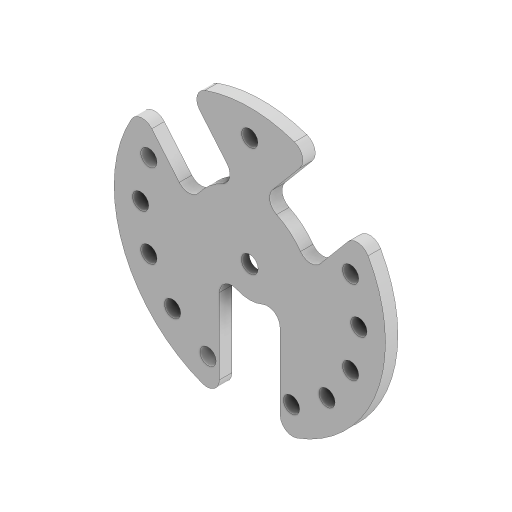
# Autodesk Inventor part: LED disk
Saved by Autodesk Inventor 2024 (Build 280153000, 153)
## iProperties
Created: 2025-04-26
Part Number: LED disk
Material: Generic
Document SubType Name: Modeling
Designer: Binara
Density: 1 g/cm^3
Appearance: Default
Author: Binara
## iProperties of the stored document LED disk_3DPrint.ipt
Created: 2025-04-26
Part Number: LED disk_3DPrint
Material: Generic
Document SubType Name: Modeling
Designer: Binara
Density: 1 g/cm^3
Appearance: Default
Author: Binara
Autodesk Inventor part; units mm, degrees
ref_plane "YZ Plane" through (0, 0, 0) normal (1, 0, 0) x (0, 1, 0)
ref_plane "XZ Plane" through (0, 0, 0) normal (0, 1, 0) x (-1, 0, 0)
ref_plane "XY Plane" through (0, 0, 0) normal (0, 0, 1) x (1, 0, 0)
sketch "Sketch1" plane through (0, 0, 0) normal (0, 0, 1) x (1, 0, 0)
  circle A0 centre (0, 0) radius 43.5
  circle A1 centre (0, 35) radius 2.6
  circle A2 centre (-13.3939, 32.3358) radius 2.6
  circle A3 centre (-24.7487, 24.7487) radius 2.6
  circle A4 centre (-32.3358, 13.3939) radius 2.6
  circle A5 centre (-35, 0) radius 2.6
  circle A6 centre (-32.3358, -13.3939) radius 2.6
  circle A7 centre (-24.7487, -24.7487) radius 2.6
  circle A8 centre (-13.3939, -32.3358) radius 2.6
  circle A9 centre (0, -35) radius 2.6
  circle A10 centre (13.3939, -32.3358) radius 2.6
  circle A11 centre (24.7487, -24.7487) radius 2.6
  circle A12 centre (32.3358, -13.3939) radius 2.6
  circle A13 centre (35, 0) radius 2.6
  circle A14 centre (32.3358, 13.3939) radius 2.6
  circle A15 centre (24.7487, 24.7487) radius 2.6
  circle A16 centre (13.3939, 32.3358) radius 2.6
  line L0 (0, 0) -> (0, -92.2535) construction
  line L1 (-9.7254, 0) -> (-9.7254, -92.2535)
  line L2 (9.7254, -92.2535) -> (9.7254, 0)
  arc A17 (9.7254, 0) -> (-9.7254, 0) centre (0, 0) ccw
  arc A18 (-9.7254, -92.2535) -> (9.7254, -92.2535) centre (0, -92.2535) ccw
  line L3 (0, 0) -> (-60.6432, 72.2718) construction
  line L4 (-7.6604, -6.4279) -> (-68.3037, 65.8439)
  line L5 (-52.9828, 78.6997) -> (7.6604, 6.4279)
  arc A19 (-7.6604, -6.4279) -> (7.6604, 6.4279) centre (0, 0) ccw
  arc A20 (-52.9828, 78.6997) -> (-68.3037, 65.8439) centre (-60.6432, 72.2718) ccw
  line L6 (0, 0) -> (65.9097, 78.5481) construction
  line L7 (-7.6604, 6.4279) -> (58.2493, 84.976)
  line L8 (73.5702, 72.1203) -> (7.6604, -6.4279)
  arc A21 (-7.6604, 6.4279) -> (7.6604, -6.4279) centre (0, 0) ccw
  arc A22 (73.5702, 72.1203) -> (58.2493, 84.976) centre (65.9097, 78.5481) ccw
  circle A23 centre (0, 0) radius 20
  point P0 (0, -46.1267)
  point P1 (-30.3216, 36.1359)
  point P2 (32.9549, 39.2741)
  point P3 (18.7939, 6.8404)
  point P4 (3.473, 19.6962)
  point P5 (19.552, 38.8583)
  point P6 (-19.552, 38.8583)
  point P7 (-3.473, 19.6962)
  point P8 (-18.7939, 6.8404)
  point P9 (-34.8728, 26.0026)
  point P10 (-9.7254, -42.3989)
  point P11 (-9.7254, -17.4762)
  point P12 (9.7254, -17.4762)
  point P13 (9.7254, -42.3989)
  point P14 (34.8728, 26.0026)
  point P15 (7.6604, -6.4279)
  point P16 (9.7254, -3.9669)
  point P17 (-9.7254, -3.9669)
  dimension "d0" = 87
  dimension "d1" = 5.2
  dimension "d2" = 35
  dimension "d5" = 360
  dimension "d7" = 140
  dimension "d8" = 140
  dimension "d9" = 10
  dimension "d10" = 10
  dimension "d11" = 40
  constraints: 24 centre point, 24 end point, 12 point on circle, 12 tangent, 3 midpoint, 3 parallel, 2 coincident, 1 vertical, 33 other
  measures "d0" diameter of A0
  measures "d1" diameter of A1
  measures "d2" distance of point (0, 0) A1.centre
  measures "d7" angle of L0 L3
  measures "d8" angle of L0 L6
  measures "d9" radius of A22
  measures "d10" radius of A20
  measures "d11" diameter of A23
extrude "Extrusion1" add sketch "Sketch1" along normal blind 4 contours A0 L2 A23 L8 | L7 A16 A23 L5 A2 A0 | A23 L2 L8 | L8 L2 A19 L5 L7 A23 | A0 L4 A23 L1 | L7 A16 | L8 A19 L2 | L7 L5 A23 | A23 L4 L1 | A2 L5 | A19 A21 L1 A17 L2 | L2 A17 L1 A21 L7 L5 A19 | L7 A21 L1 L4 A23 L5 | L1 A21 L4 picked at (13.6821, 33.106) picked at (-12.7209, 31.8549)
sketch "Sketch2" plane through (0, 0, 0) normal (0, 0, -1) x (-1, 0, 0)
  circle A0 centre (0, 0) radius 7.65
  dimension "d14" = 15.3
  constraints: 1 centre point, 1 coincident
  measures "d14" diameter of A0
extrude "Extrusion2" cut sketch "Sketch2" against normal blind 1.5
sketch "Sketch3" plane through (0, 0, 1.5) normal (0, 0, -1) x (-1, 0, 0)
  circle A0 centre (0, 0) radius 2.7
  dimension "d17" = 5.4
  constraints: 1 centre point, 1 coincident
  measures "d17" diameter of A0
extrude "Extrusion3" cut sketch "Sketch3" against normal up to surface (2.5 mm away)
fillet "Fillet1" radius 4 12 edges at (9.7254, -3.9669, 2) (-9.7254, -3.9669, 2) (3.473, 19.6962, 2) (18.7939, 6.8404, 2) (-18.7939, 6.8404, 2) (-3.473, 19.6962, 2) (34.8728, 26.0026, 2) (19.552, 38.8583, 2) (-19.552, 38.8583, 2) (-34.8728, 26.0026, 2) (-9.7254, -42.3989, 2) (9.7254, -42.3989, 2)
equation "\"d10\" = d9"
body "Solid1"
